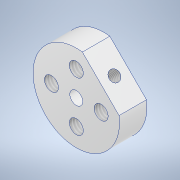
# Autodesk Inventor part: Wheel Hub
Saved by Autodesk Inventor 2022 (Build 260153000, 153)
## iProperties
Created: 2022-08-21
Part Number: Wheel Hub
Material: Aluminum 6061
Document SubType Name: Modeling
Designer: Nick
Density: 2.7 g/cm^3
Appearance: Aluminum - Flat
Mass: 3.97923 g
Surface Area: 12.9976 cm^2
Volume: 1.47379 cm^3
Author: Nick
Autodesk Inventor part; units mm, degrees
ref_plane "YZ Plane" through (0, 0, 0) normal (1, 0, 0) x (0, 1, 0)
ref_plane "XZ Plane" through (0, 0, 0) normal (0, 1, 0) x (-1, 0, 0)
ref_plane "XY Plane" through (0, 0, 0) normal (0, 0, 1) x (1, 0, 0)
sketch "Sketch1" plane through (0, 0, 0) normal (0, 0, 1) x (1, 0, 0)
  circle A0 centre (0, 0) radius 1.5
  circle A1 centre (0, 0) radius 10
  dimension "d0" = 3
  dimension "d1" = 20
  constraints: 2 centre point, 2 coincident
  measures "d0" diameter of A0
  measures "d1" diameter of A1
extrude "Extrusion1" add sketch "Sketch1" along normal blind 6.35
sketch "Sketch2" plane through (0, 0, 6.35) normal (0, 0, 1) x (1, 0, 0)
  circle A0 centre (0, 0) radius 10 projected
  circle A1 centre (0, 0) radius 1.5 projected
  line L0 (-1.7564, 1.5) -> (1.7564, 1.5) construction
  line L1 (-1.2885, 10) -> (1.2885, 10) construction
  point P0 (0, 5.75)
  point P1 (0, 10)
  point P2 (0, 1.5)
  dimension "d26" = 4.25
  dimension "d27" = 4.25
  constraints: 4 end point, 3 vertical alignment, 2 horizontal, 2 midpoint, 2 tangent
  measures "d26" distance from line of point (0, 5.75) L1
  measures "d27" distance from line of L0 point (0, 5.75)
hole "Hole1" at (0, 5.75, 6.35) direction (0, 0, -1) diameter 3.242 end through all thread size "M4x0.7" class "6H" standard "ANSI Metric M Profile"
pattern_circular "Circular Pattern1" count 4 over 360 about axis through (0, 0, 0) along (0, 0, 1) of "Hole1"
sketch "Sketch3" plane through (0, 0, 6.35) normal (0, 0, 1) x (1, 0, 0)
  line L0 (9.8995, 1.4142) -> (1.4142, 9.8995)
  line L1 (0, 0) -> (5.6569, 5.6569)
  line L2 (0, 0) -> (0, 3.1175)
  circle A0 centre (5.75, 0) radius 1.621 projected
  circle A1 centre (0, -5.75) radius 1.621 projected
  circle A2 centre (-5.75, 0) radius 1.621 projected
  circle A3 centre (0, 5.75) radius 1.621 projected
  circle A4 centre (0, 0) radius 10 projected
  circle A5 centre (0, 0) radius 1.5 projected
  circle A6 centre (0, 0) radius 10 projected
  point P0 (1.4142, 9.8995)
  point P1 (9.8995, 1.4142)
  point P2 (-0.5834, 9.983)
  point P3 (-9.983, 0.5834)
  dimension "d15" = 45
  dimension "d16" = 8
  constraints: 6 end point, 1 midpoint, 1 perpendicular, 1 point on circle, 1 vertical
  measures "d15" angle of L1 L2
  measures "d16" distance of L1.start L1.end
extrude "Extrusion2" cut sketch "Sketch3" against normal blind 8 contours L0 A4 picked at (3.52, 8.3093)
sketch "Sketch4" plane through (9.8995, 1.4142, 0) normal (0.7071068, 0.7071068, 0) x (-0.7071068, 0.7071068, 0)
  line L0 (4.5, 6.35) -> (7.5, 6.35) projected
  line L1 (4.5, 0) -> (7.5, 0) projected
  line L2 (4.5, 6.35) -> (7.5, 6.35) construction
  line L3 (3.5551, 0) -> (0.3131, 0) construction
  line L4 (7.5, 6.35) -> (3.5551, 6.35) construction
  line L5 (3.5551, 6.35) -> (3.5551, 0) construction
  line L6 (3.5551, 0) -> (7.5, 0) construction
  line L7 (7.5, 0) -> (7.5, 6.35) construction
  point P0 (6, 0)
  point P1 (6, 3.175)
  point P2 (7.5, 3.175)
  point P3 (6, 0)
  constraints: 8 end point, 2 midpoint, 2 parallel, 1 horizontal, 1 horizontal alignment, 1 perpendicular, 1 vertical alignment
hole "Hole2" at (5.6569, 5.6569, 3.175) direction (-0.7071068, -0.7071068, 0) diameter 2.459 depth 8.8 tip angle 118 thread size "M3x0.5" class "6H" standard "ANSI Metric M Profile"
equation "\"d26\" = d27"
body "Solid1"
